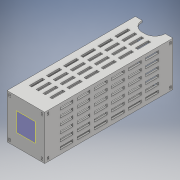
# Autodesk Inventor part: battery_cage
Saved by Autodesk Inventor 2018 (Build 220112000, 112)
## iProperties
Created: 2019-11-14
Part Number: battery_cage
Material: Generic
Document SubType Name: Modeling
Designer: bitbots
Density: 1 g/cm^3
Appearance: Default
Author: bitbots
Autodesk Inventor part; units mm, degrees
ref_plane "YZ Plane" through (0, 0, 0) normal (1, 0, 0) x (0, 1, 0)
ref_plane "XZ Plane" through (0, 0, 0) normal (0, 1, 0) x (-1, 0, 0)
ref_plane "XY Plane" through (0, 0, 0) normal (0, 0, 1) x (1, 0, 0)
ref_plane "Work Plane2" through (0, 2.5, 0) normal (0, 1, 0) x (1, 0, 0)
sketch "Sketch7" plane through (0, 2.5, 0) normal (0, 1, 0) x (1, 0, 0)
  line L0 (-22, -26) -> (22, -26)
  line L1 (22, -26) -> (22, 26)
  line L2 (22, 26) -> (-22, 26)
  line L3 (-22, 26) -> (-22, -26)
  line L4 (-22, -26) -> (22, 26) construction
  line L5 (22, -26) -> (-22, 26) construction
  line L6 (20, -24) -> (-20, -24)
  line L7 (-20, -24) -> (-20, 24)
  line L8 (-20, 24) -> (20, 24)
  line L9 (20, 24) -> (20, -24)
  line L10 (20, -24) -> (-20, 24) construction
  line L11 (-20, -24) -> (20, 24) construction
  point P0 (0, 0)
  dimension "d30" = 44
  dimension "d31" = 52
  dimension "d34" = 40
  dimension "d35" = 48
  constraints: 24 end point, 4 midpoint, 4 parallel, 2 horizontal, 2 perpendicular
  measures "d30" distance of L2.end L1.end
  measures "d31" distance of L1.end L0.end
  measures "d34" distance of L7.end L8.end
  measures "d35" distance of L6.end L7.end
extrude "Extrusion9" add sketch "Sketch7" along normal blind 3 contours L6 L7 L8 L9
sketch "Sketch8" plane through (0, 2.5, 0) normal (0, -1, 0) x (1, 0, 0)
  line L0 (20, 24) -> (-20, 24)
  line L1 (-20, 24) -> (-20, -24)
  line L2 (-20, -24) -> (20, -24)
  line L3 (20, -24) -> (20, 24)
  line L4 (20, 24) -> (-20, -24) construction
  line L5 (-20, 24) -> (20, -24) construction
  line L6 (22, 26) -> (-22, 26)
  line L7 (-22, 26) -> (-22, -26)
  line L8 (-22, -26) -> (22, -26)
  line L9 (22, -26) -> (22, 26)
  line L10 (22, 26) -> (-22, -26) construction
  line L11 (-22, 26) -> (22, -26) construction
  point P0 (0, 0)
  dimension "d40" = 40
  dimension "d41" = 48
  dimension "d42" = 44
  dimension "d43" = 52
  constraints: 24 end point, 4 midpoint, 4 parallel, 2 horizontal, 2 perpendicular
  measures "d40" distance of L2.end L1.end
  measures "d41" distance of L1.end L0.end
  measures "d42" distance of L8.end L7.end
  measures "d43" distance of L7.end L6.end
extrude "Extrusion10" add sketch "Sketch8" against normal blind 150
sketch "Sketch11" plane through (0, 2.5, 0) normal (0, -1, 0) x (1, 0, 0)
  line L0 (-20, -24) -> (-18, -24)
  line L1 (-18, -24) -> (-18, -21)
  line L2 (-18, -21) -> (-20, -21)
  line L3 (-20, -21) -> (-20, -24)
  line L4 (-20, 24) -> (-18, 24)
  line L5 (-18, 24) -> (-18, 21)
  line L6 (-18, 21) -> (-20, 21)
  line L7 (-20, 21) -> (-20, 24)
  line L8 (22, 26) -> (-22, 26) construction
  line L9 (0, 26) -> (0, -26) construction
  line L10 (-22, -26) -> (22, -26) construction
  line L11 (20, -24) -> (18, -24)
  line L12 (18, -24) -> (18, -21)
  line L13 (18, -21) -> (20, -21)
  line L14 (20, -21) -> (20, -24)
  line L15 (20, 24) -> (18, 24)
  line L16 (18, 24) -> (18, 21)
  line L17 (18, 21) -> (20, 21)
  line L18 (20, 21) -> (20, 24)
  point P0 (0, 0)
  dimension "d73" = 2
  dimension "d74" = 3
  dimension "d75" = 2
  dimension "d76" = 3
  constraints: 34 end point, 8 symmetric about line, 4 parallel, 2 horizontal, 2 midpoint, 2 perpendicular
  measures "d73" distance of L2.end L1.end
  measures "d74" distance of L1.end L0.end
  measures "d75" distance of L5.end L6.end
  measures "d76" distance of L4.end L5.end
sketch "Sketch12" plane through (-22, 2.5, -26) normal (-1, 0, 0) x (0, 0, 1)
  line L0 (2, 3) -> (2, 150) projected
  line L1 (2, 3) -> (5, 3)
  line L2 (5, 3) -> (5, 5)
  line L3 (5, 5) -> (2, 5)
  line L4 (2, 5) -> (2, 3)
  line L5 (50, 3) -> (50, 150) projected
  line L6 (50, 3) -> (47, 3)
  line L7 (47, 3) -> (47, 5)
  line L8 (47, 5) -> (50, 5)
  line L9 (50, 5) -> (50, 3)
  line L10 (2, 148) -> (5, 148)
  line L11 (5, 148) -> (5, 146)
  line L12 (5, 146) -> (2, 146)
  line L13 (2, 146) -> (2, 148)
  line L14 (2, 148) -> (50, 148) projected
  line L15 (50, 148) -> (47, 148)
  line L16 (47, 148) -> (47, 146)
  line L17 (47, 146) -> (50, 146)
  line L18 (50, 146) -> (50, 148)
  line L19 (0, 0) -> (52, 0) construction
  line L20 (0, 150) -> (52, 150) construction
  line L21 (48, 0) -> (48, 150) construction
  line L22 (5, 18) -> (7.5, 18)
  line L23 (5, 18) -> (8, 18)
  line L24 (8, 18) -> (8, 33)
  line L25 (8, 33) -> (5, 33)
  line L26 (5, 33) -> (5, 18)
  line L27 (5, 38) -> (7.5, 38)
  line L28 (5, 38) -> (8, 38)
  line L29 (8, 38) -> (8, 53)
  line L30 (5, 53) -> (5, 38)
  line L31 (8, 53) -> (5, 53)
  line L32 (5, 58) -> (7.5, 58)
  line L33 (5, 58) -> (8, 58)
  line L34 (8, 58) -> (8, 73)
  line L35 (5, 73) -> (5, 58)
  line L36 (8, 73) -> (5, 73)
  line L37 (5, 78) -> (7.5, 78)
  line L38 (5, 78) -> (8, 78)
  line L39 (8, 78) -> (8, 93)
  line L40 (5, 93) -> (5, 78)
  line L41 (8, 93) -> (5, 93)
  line L42 (5, 98) -> (7.5, 98)
  line L43 (5, 98) -> (8, 98)
  line L44 (8, 98) -> (8, 113)
  line L45 (5, 113) -> (5, 98)
  line L46 (8, 113) -> (5, 113)
  line L47 (5, 118) -> (7.5, 118)
  line L48 (5, 118) -> (8, 118)
  line L49 (8, 118) -> (8, 133)
  line L50 (5, 133) -> (5, 118)
  line L51 (8, 133) -> (5, 133)
  line L52 (13, 18) -> (15.5, 18)
  line L53 (13, 18) -> (16, 18)
  line L54 (16, 18) -> (16, 33)
  line L55 (13, 33) -> (13, 18)
  line L56 (16, 33) -> (13, 33)
  line L57 (13, 38) -> (15.5, 38)
  line L58 (13, 38) -> (16, 38)
  line L59 (16, 38) -> (16, 53)
  line L60 (13, 53) -> (13, 38)
  line L61 (16, 53) -> (13, 53)
  line L62 (13, 58) -> (15.5, 58)
  line L63 (13, 58) -> (16, 58)
  line L64 (16, 58) -> (16, 73)
  line L65 (13, 73) -> (13, 58)
  line L66 (16, 73) -> (13, 73)
  line L67 (13, 78) -> (15.5, 78)
  line L68 (13, 78) -> (16, 78)
  line L69 (16, 78) -> (16, 93)
  line L70 (13, 93) -> (13, 78)
  line L71 (16, 93) -> (13, 93)
  line L72 (13, 98) -> (15.5, 98)
  line L73 (13, 98) -> (16, 98)
  line L74 (16, 98) -> (16, 113)
  line L75 (13, 113) -> (13, 98)
  line L76 (16, 113) -> (13, 113)
  line L77 (13, 118) -> (15.5, 118)
  line L78 (13, 118) -> (16, 118)
  line L79 (16, 118) -> (16, 133)
  line L80 (13, 133) -> (13, 118)
  line L81 (16, 133) -> (13, 133)
  line L82 (21, 18) -> (23.5, 18)
  line L83 (21, 18) -> (24, 18)
  line L84 (24, 18) -> (24, 33)
  line L85 (21, 33) -> (21, 18)
  line L86 (24, 33) -> (21, 33)
  line L87 (21, 38) -> (23.5, 38)
  line L88 (21, 38) -> (24, 38)
  line L89 (24, 38) -> (24, 53)
  line L90 (21, 53) -> (21, 38)
  line L91 (24, 53) -> (21, 53)
  line L92 (21, 58) -> (23.5, 58)
  line L93 (21, 58) -> (24, 58)
  line L94 (24, 58) -> (24, 73)
  line L95 (21, 73) -> (21, 58)
  line L96 (24, 73) -> (21, 73)
  line L97 (21, 78) -> (23.5, 78)
  line L98 (21, 78) -> (24, 78)
  line L99 (24, 78) -> (24, 93)
  line L100 (21, 93) -> (21, 78)
  line L101 (24, 93) -> (21, 93)
  line L102 (21, 98) -> (23.5, 98)
  line L103 (21, 98) -> (24, 98)
  line L104 (24, 98) -> (24, 113)
  line L105 (21, 113) -> (21, 98)
  line L106 (24, 113) -> (21, 113)
  line L107 (21, 118) -> (23.5, 118)
  line L108 (21, 118) -> (24, 118)
  line L109 (24, 118) -> (24, 133)
  line L110 (21, 133) -> (21, 118)
  line L111 (24, 133) -> (21, 133)
  line L112 (29, 18) -> (31.5, 18)
  line L113 (29, 18) -> (32, 18)
  line L114 (32, 18) -> (32, 33)
  line L115 (29, 33) -> (29, 18)
  line L116 (32, 33) -> (29, 33)
  line L117 (29, 38) -> (31.5, 38)
  line L118 (29, 38) -> (32, 38)
  line L119 (32, 38) -> (32, 53)
  line L120 (29, 53) -> (29, 38)
  line L121 (32, 53) -> (29, 53)
  line L122 (29, 58) -> (31.5, 58)
  line L123 (29, 58) -> (32, 58)
  line L124 (32, 58) -> (32, 73)
  line L125 (29, 73) -> (29, 58)
  line L126 (32, 73) -> (29, 73)
  line L127 (29, 78) -> (31.5, 78)
  line L128 (29, 78) -> (32, 78)
  line L129 (32, 78) -> (32, 93)
  line L130 (29, 93) -> (29, 78)
  line L131 (32, 93) -> (29, 93)
  line L132 (29, 98) -> (31.5, 98)
  line L133 (29, 98) -> (32, 98)
  line L134 (32, 98) -> (32, 113)
  line L135 (29, 113) -> (29, 98)
  line L136 (32, 113) -> (29, 113)
  line L137 (29, 118) -> (31.5, 118)
  line L138 (29, 118) -> (32, 118)
  line L139 (32, 118) -> (32, 133)
  line L140 (29, 133) -> (29, 118)
  line L141 (32, 133) -> (29, 133)
  line L142 (37, 18) -> (39.5, 18)
  line L143 (37, 18) -> (40, 18)
  line L144 (40, 18) -> (40, 33)
  line L145 (37, 33) -> (37, 18)
  line L146 (40, 33) -> (37, 33)
  line L147 (37, 38) -> (39.5, 38)
  line L148 (37, 38) -> (40, 38)
  line L149 (40, 38) -> (40, 53)
  line L150 (37, 53) -> (37, 38)
  line L151 (40, 53) -> (37, 53)
  line L152 (37, 58) -> (39.5, 58)
  line L153 (37, 58) -> (40, 58)
  line L154 (40, 58) -> (40, 73)
  line L155 (37, 73) -> (37, 58)
  line L156 (40, 73) -> (37, 73)
  line L157 (37, 78) -> (39.5, 78)
  line L158 (37, 78) -> (40, 78)
  line L159 (40, 78) -> (40, 93)
  line L160 (37, 93) -> (37, 78)
  line L161 (40, 93) -> (37, 93)
  line L162 (37, 98) -> (39.5, 98)
  line L163 (37, 98) -> (40, 98)
  line L164 (40, 98) -> (40, 113)
  line L165 (37, 113) -> (37, 98)
  line L166 (40, 113) -> (37, 113)
  line L167 (37, 118) -> (39.5, 118)
  line L168 (37, 118) -> (40, 118)
  line L169 (40, 118) -> (40, 133)
  line L170 (37, 133) -> (37, 118)
  line L171 (40, 133) -> (37, 133)
  line L172 (45, 18) -> (47.5, 18)
  line L173 (45, 18) -> (48, 18)
  line L174 (48, 18) -> (48, 33)
  line L175 (45, 33) -> (45, 18)
  line L176 (48, 33) -> (45, 33)
  line L177 (45, 38) -> (47.5, 38)
  line L178 (45, 38) -> (48, 38)
  line L179 (48, 38) -> (48, 53)
  line L180 (45, 53) -> (45, 38)
  line L181 (48, 53) -> (45, 53)
  line L182 (45, 58) -> (47.5, 58)
  line L183 (45, 58) -> (48, 58)
  line L184 (48, 58) -> (48, 73)
  line L185 (45, 73) -> (45, 58)
  line L186 (48, 73) -> (45, 73)
  line L187 (45, 78) -> (47.5, 78)
  line L188 (45, 78) -> (48, 78)
  line L189 (48, 78) -> (48, 93)
  line L190 (45, 93) -> (45, 78)
  line L191 (48, 93) -> (45, 93)
  line L192 (45, 98) -> (47.5, 98)
  line L193 (45, 98) -> (48, 98)
  line L194 (48, 98) -> (48, 113)
  line L195 (45, 113) -> (45, 98)
  line L196 (48, 113) -> (45, 113)
  line L197 (45, 118) -> (47.5, 118)
  line L198 (45, 118) -> (48, 118)
  line L199 (48, 118) -> (48, 133)
  line L200 (45, 133) -> (45, 118)
  line L201 (48, 133) -> (45, 133)
  dimension "d79" = 3
  dimension "d80" = 2
  dimension "d81" = 3
  dimension "d82" = 2
  dimension "d83" = 3
  dimension "d84" = 2
  dimension "d85" = 3
  dimension "d92" = 13
  dimension "d93" = 3
  dimension "d94" = 15
  dimension "d95" = 3
  dimension "d108" = 20
  dimension "d111" = 8
  constraints: 394 end point, 10 parallel, 7 horizontal, 5 perpendicular, 2 collinear, 2 vertical, 1 point on line, 348 other
  measures "d79" distance of L3.end L2.end
  measures "d80" distance of L2.end L1.end
  measures "d81" distance of L7.end L8.end
  measures "d82" distance of L6.end L7.end
  measures "d83" distance of L11.end L12.end
  measures "d84" distance of L10.end L11.end
  measures "d85" distance between parallel lines of L18 L16
  measures "d92" distance between parallel lines of L3 L22
  measures "d93" distance of L25.end L24.end
  measures "d94" distance of L24.end L23.end
  measures "d95" distance between parallel lines of L26 L0
  measures "d108" distance of L23.end L28.end
  measures "d111" distance of L23.end L53.end
extrude "Extrusion15" cut sketch "Sketch11" against normal blind 10
extrude "Extrusion16" cut sketch "Sketch12" against normal through all
sketch "Sketch13" plane through (22, 2.5, -26) normal (0, 0, -1) x (-1, 0, 0)
  line L0 (0, 0) -> (0, 150) construction
  line L1 (44, 0) -> (0, 0) construction
  line L2 (44, 0) -> (44, 150) construction
  line L3 (44, 150) -> (0, 150) construction
  line L4 (42, 148) -> (2, 148) construction
  line L5 (0, 18) -> (44, 18) construction
  line L6 (44, 0) -> (44, 150) construction
  line L7 (0, 0) -> (44, 0) construction
  line L8 (9, 0) -> (9, 150) construction
  line L9 (44, 150) -> (0, 150) construction
  line L10 (9, 18) -> (12, 18)
  line L11 (12, 18) -> (12, 33)
  line L12 (12, 33) -> (9, 33)
  line L13 (9, 33) -> (9, 18)
  line L14 (9, 38) -> (12, 38)
  line L15 (12, 38) -> (12, 53)
  line L16 (12, 53) -> (9, 53)
  line L17 (9, 53) -> (9, 38)
  line L18 (9, 58) -> (12, 58)
  line L19 (12, 58) -> (12, 73)
  line L20 (12, 73) -> (9, 73)
  line L21 (9, 73) -> (9, 58)
  line L22 (9, 78) -> (12, 78)
  line L23 (12, 78) -> (12, 93)
  line L24 (12, 93) -> (9, 93)
  line L25 (9, 93) -> (9, 78)
  line L26 (9, 98) -> (12, 98)
  line L27 (12, 98) -> (12, 113)
  line L28 (12, 113) -> (9, 113)
  line L29 (9, 113) -> (9, 98)
  line L30 (9, 118) -> (12, 118)
  line L31 (12, 118) -> (12, 133)
  line L32 (12, 133) -> (9, 133)
  line L33 (9, 133) -> (9, 118)
  line L34 (17, 18) -> (20, 18)
  line L35 (20, 18) -> (20, 33)
  line L36 (20, 33) -> (17, 33)
  line L37 (17, 33) -> (17, 18)
  line L38 (17, 38) -> (20, 38)
  line L39 (20, 38) -> (20, 53)
  line L40 (20, 53) -> (17, 53)
  line L41 (17, 53) -> (17, 38)
  line L42 (17, 58) -> (20, 58)
  line L43 (20, 58) -> (20, 73)
  line L44 (20, 73) -> (17, 73)
  line L45 (17, 73) -> (17, 58)
  line L46 (17, 78) -> (20, 78)
  line L47 (20, 78) -> (20, 93)
  line L48 (20, 93) -> (17, 93)
  line L49 (17, 93) -> (17, 78)
  line L50 (17, 98) -> (20, 98)
  line L51 (20, 98) -> (20, 113)
  line L52 (20, 113) -> (17, 113)
  line L53 (17, 113) -> (17, 98)
  line L54 (17, 118) -> (20, 118)
  line L55 (20, 118) -> (20, 133)
  line L56 (20, 133) -> (17, 133)
  line L57 (17, 133) -> (17, 118)
  line L58 (25, 18) -> (28, 18)
  line L59 (28, 18) -> (28, 33)
  line L60 (28, 33) -> (25, 33)
  line L61 (25, 33) -> (25, 18)
  line L62 (25, 38) -> (28, 38)
  line L63 (28, 38) -> (28, 53)
  line L64 (28, 53) -> (25, 53)
  line L65 (25, 53) -> (25, 38)
  line L66 (25, 58) -> (28, 58)
  line L67 (28, 58) -> (28, 73)
  line L68 (28, 73) -> (25, 73)
  line L69 (25, 73) -> (25, 58)
  line L70 (25, 78) -> (28, 78)
  line L71 (28, 78) -> (28, 93)
  line L72 (28, 93) -> (25, 93)
  line L73 (25, 93) -> (25, 78)
  line L74 (25, 98) -> (28, 98)
  line L75 (28, 98) -> (28, 113)
  line L76 (28, 113) -> (25, 113)
  line L77 (25, 113) -> (25, 98)
  line L78 (25, 118) -> (28, 118)
  line L79 (28, 118) -> (28, 133)
  line L80 (28, 133) -> (25, 133)
  line L81 (25, 133) -> (25, 118)
  line L82 (33, 18) -> (36, 18)
  line L83 (36, 18) -> (36, 33)
  line L84 (36, 33) -> (33, 33)
  line L85 (33, 33) -> (33, 18)
  line L86 (33, 38) -> (36, 38)
  line L87 (36, 38) -> (36, 53)
  line L88 (36, 53) -> (33, 53)
  line L89 (33, 53) -> (33, 38)
  line L90 (33, 58) -> (36, 58)
  line L91 (36, 58) -> (36, 73)
  line L92 (36, 73) -> (33, 73)
  line L93 (33, 73) -> (33, 58)
  line L94 (33, 78) -> (36, 78)
  line L95 (36, 78) -> (36, 93)
  line L96 (36, 93) -> (33, 93)
  line L97 (33, 93) -> (33, 78)
  line L98 (33, 98) -> (36, 98)
  line L99 (36, 98) -> (36, 113)
  line L100 (36, 113) -> (33, 113)
  line L101 (33, 113) -> (33, 98)
  line L102 (33, 118) -> (36, 118)
  line L103 (36, 118) -> (36, 133)
  line L104 (36, 133) -> (33, 133)
  line L105 (33, 133) -> (33, 118)
  line L106 (36, 133) -> (36, 150) construction
  line L107 (9, 150) -> (36, 150) construction
  line L108 (36, 150) -> (36, 138) construction
  line L109 (36, 138) -> (9, 138) construction
  line L110 (9, 138) -> (9, 150) construction
  line L111 (9, 150) -> (36, 150)
  line L112 (36, 150) -> (36, 138)
  line L113 (36, 138) -> (9, 138)
  line L114 (9, 138) -> (9, 150)
  line L115 (0, 150) -> (44, 150) construction
  line L116 (36, 138) -> (21, 138) construction
  line L117 (21, 150) -> (32, 150) construction
  line L118 (44, 150) -> (0, 150) construction
  line L119 (22.5, 150) -> (22.5, 138) construction
  line L120 (21, 150) -> (21, 138) construction
  line L121 (24, 150) -> (24, 138) construction
  circle A0 centre (21, 150) radius 12
  circle A1 centre (24, 150) radius 12
  line L122 (21, 150) -> (24, 150) construction
  line L123 (21, 138) -> (24, 138) construction
  line L124 (21, 150) -> (24, 150)
  line L125 (24, 150) -> (24, 138)
  line L126 (24, 138) -> (21, 138)
  line L127 (21, 138) -> (21, 150)
  dimension "d117" = 18
  dimension "d118" = 9
  dimension "d119" = 3
  dimension "d120" = 15
  dimension "d123" = 20
  dimension "d126" = 8
  dimension "d131" = 12
  dimension "d147" = 27
  dimension "d148" = 13.5
  dimension "d149" = 12
  constraints: 240 end point, 10 parallel, 10 point on line, 8 perpendicular, 6 horizontal, 3 collinear, 3 vertical, 2 coincident, 2 horizontal alignment, 2 symmetric about line, 1 midpoint, 190 other
  measures "d117" distance between parallel lines of L1 L5
  measures "d118" distance between parallel lines of L8 L0
  measures "d119" distance of L12.end L11.end
  measures "d120" distance of L11.end L10.end
  measures "d123" distance of L10.start L14.start
  measures "d126" distance of L10.start L34.start
  measures "d131" distance of L107.end L108.end
  measures "d147" distance of L108.end L113.end
  measures "d148" distance between parallel lines of L114 L119
  measures "d149" distance between parallel lines of L8 L120
extrude "Extrusion19" cut sketch "Sketch13" against normal through all contours L13 L12 L11 L10 | L17 L16 L15 L14 | L21 L20 L19 L18 | L25 L24 L23 L22 | L29 L28 L27 L26 | L33 L32 L31 L30 | L37 L36 L35 L34 | L41 L40 L39 L38 | L45 L44 L43 L42 | L49 L48 L47 L46 | L53 L52 L51 L50 | L57 L56 L55 L54 | L61 L60 L59 L58 | L65 L64 L63 L62 | L69 L68 L67 L66 | L73 L72 L71 L70 | L77 L76 L75 L74 | L81 L80 L79 L78 | L85 L84 L83 L82 | L89 L88 L87 L86 | L93 L92 L91 L90 | L97 L96 L95 L94 | L101 L100 L99 L98 | L105 L104 L103 L102 | L111 A1 A0 | L127 A1 L111 | L111 L125 A0 A1 L127 | L111 A0 L125 | A1 L127 A0 L111 | L111 A0 A1 | A1 A0 L127 | A0 A1 L111 | L111 A1 L125 A0 | L125 A1 A0 | A1 L113 A0
equation "\"d30\" = max_width"
equation "\"d31\" = max_heigth"
equation "\"d34\" = bat_width"
equation "\"d35\" = bat_heigth"
equation "\"d38\" = default"
equation "\"d40\" = bat_width"
equation "\"d41\" = bat_heigth"
equation "\"d42\" = max_width"
equation "\"d43\" = max_heigth"
equation "\"d44\" = robot_width"
equation "\"bat_width\" = 40"
equation "\"bat_heigth\" = 48"
equation "\"max_heigth\" = 52"
equation "\"max_width\" = 44"
equation "\"robot_width\" = 150"
equation "\"default\" = 3"
body "Solid6"
